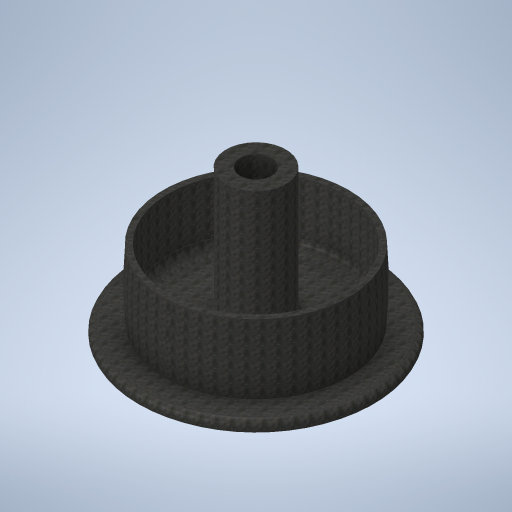
# Autodesk Inventor part: kumar_Pully
Saved by Autodesk Inventor 2024 (Build 280153000, 153)
## iProperties
Created: 2024-10-10
Part Number: kumar_Pully
Material: Steel
Document SubType Name: Modeling
Designer: NK
Density: 7.85 g/cm^3
Appearance: Plate
Mass: 3.17255e+07 g
Surface Area: 480361 cm^2
Volume: 4.04147e+06 cm^3
Author: itsimg
Autodesk Inventor part; units mm, degrees
ref_plane "YZ Plane" through (0, 0, 0) normal (1, 0, 0) x (0, 1, 0)
ref_plane "XZ Plane" through (0, 0, 0) normal (0, 1, 0) x (-1, 0, 0)
ref_plane "XY Plane" through (0, 0, 0) normal (0, 0, 1) x (1, 0, 0)
sketch "Sketch1" plane through (0, 0, 0) normal (1, 0, 0) x (0, 1, 0)
  line L0 (365.6546, 253.56) -> (365.6546, 761.56)
  line L1 (365.6546, 761.56) -> (365.6546, 761.56)
  line L2 (441.8546, 837.76) -> (441.8546, 1968.06)
  line L3 (645.0546, 1968.06) -> (645.0546, 1663.8825)
  line L4 (1711.8546, 1670.0758) -> (1711.8546, 710.76)
  line L5 (899.0546, 710.76) -> (2727.8546, 710.76)
  line L6 (2727.8546, 710.76) -> (2727.8546, 253.56)
  line L7 (365.6546, 253.56) -> (2219.8546, 253.56)
  line L8 (2727.8546, 253.56) -> (2219.8546, 253.56)
  line L9 (2727.8546, 494.86) -> (2219.8546, 494.86)
  line L10 (2219.8546, 253.56) -> (2219.8546, 494.86)
  arc A0 (645.0546, 1968.06) -> (441.8546, 1968.06) centre (543.4546, 1968.06) ccw
  line L11 (899.0546, 1587.06) -> (1711.8546, 1587.06)
  line L12 (746.6546, 1434.66) -> (746.6546, 863.16)
  arc A1 (899.0546, 1587.06) -> (746.6546, 1434.66) centre (899.0546, 1434.66) ccw
  arc A2 (746.6546, 863.16) -> (899.0546, 710.76) centre (899.0546, 863.16) ccw
  arc A3 (1711.8546, 1670.0758) -> (645.0546, 1663.8825) centre (1215.1888, -4660.471) ccw
  arc A4 (365.6546, 761.56) -> (441.8546, 837.76) centre (365.6546, 837.76) ccw
  point P0 (0, 0)
  point P1 (543.4546, 2069.66)
  point P2 (1178.3243, 1689.422)
  dimension "d0" = 914.4
  dimension "d3" = 1016
  dimension "d5" = 2362.2
  dimension "d6" = 1854.2
  dimension "d8" = 76.2
  dimension "d10" = 203.2
  dimension "d11" = 482.6
  dimension "d12" = 3632.2
  dimension "d13" = 2667
  dimension "d14" = 304.8
  dimension "d15" = 152.4
  dimension "d18" = 6350
  dimension "d19" = 2871.724
  dimension "d20" = 365.6546
  dimension "d21" = 253.56
  dimension "d23" = 76.2
  dimension "d26" = 2833.0317
  dimension "d31" = 1270
  constraints: 26 end point, 12 point on circle, 8 tangent, 6 vertical, 5 centre point, 5 horizontal, 3 point on line, 2 perpendicular, 1 equal radius
  measures "d0" diameter of L5 L8
  measures "d3" diameter of L1 L8
  measures "d5" distance between parallel lines of L6 L0
  measures "d6" distance from line of L0 L7.end
  measures "d8" distance between parallel lines of L2 L0
  measures "d10" distance between parallel lines of L3 L2
  measures "d11" diameter of L9 L8
  measures "d12" diameter of point (543.455, 2069.66) L8
  measures "d13" diameter of L11 L8
  measures "d14" distance between parallel lines of L12 L2
  measures "d15" radius of A1
  measures "d18" radius of A3
  measures "d19" diameter of point (1178.324, 1689.422) L8
  measures "d20" horizontal distance of point (0, 0) L0.start
  measures "d21" vertical distance of point (0, 0) L0.start
  measures "d23" radius of A4
  measures "d26" diameter of L4.start L8
  measures "d31" distance between parallel lines of L2 L4
revolve "Revolution1" add sketch "Sketch1" angle 360 about axis through (0, 2727.8546, 253.56) along (0, -1, 0) contours L0 A4 L2 A0 L3 A3 L4 L11 A1 L12 A2 L5 L6 L9 L10 L7
sketch "Sketch2" plane through (0, 365.6546, 253.56) normal (0, -1, 0) x (1, 0, 0)
  circle A0 centre (0, 0) radius 241.3 projected
  circle A1 centre (0, 0) radius 355.6
  dimension "d28" = 711.2
  constraints: 1 centre point, 1 coincident
  measures "d28" diameter of A1
extrude "Extrusion1" cut sketch "Sketch2" against normal blind 1854.2 contours A0 | A1
body "Solid1"
